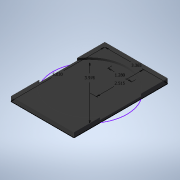
# Autodesk Inventor part: 100mm wafer wellplate
Saved by Autodesk Inventor 2020 (Build 240168000, 168)
## iProperties
Created: 2022-04-03
Part Number: 100mm wafer wellplate
Material: Generic
Document SubType Name: Modeling
Designer: Beaucage
Density: 1 g/cm^3
Appearance: Default
Author: Beaucage
Autodesk Inventor part; units mm, degrees
ref_plane "YZ Plane" through (0, 0, 0) normal (1, 0, 0) x (0, 1, 0)
ref_plane "XZ Plane" through (0, 0, 0) normal (0, 1, 0) x (-1, 0, 0)
ref_plane "XY Plane" through (0, 0, 0) normal (0, 0, 1) x (1, 0, 0)
sketch "Sketch1" plane through (0, 0, 0) normal (0, 1, 0) x (-1, 0, 0)
  line L0 (0, 0) -> (85.48, 0)
  line L1 (85.48, 0) -> (85.48, -127.76)
  line L2 (85.48, -127.76) -> (0, -127.76)
  line L3 (0, -127.76) -> (0, 0)
  line L4 (42.74, -127.76) -> (42.74, -63.879)
  circle A0 centre (42.1561, -63.879) radius 50.5
  line L5 (26.485, -111.163) -> (58.985, -111.1664)
  line L6 (42.74, -63.879) -> (42.7347, -113.879)
  point P0 (85.48, -37.9311)
  point P1 (85.48, -89.8269)
  point P2 (0, -91.6839)
  point P3 (0, -36.0741)
  point P4 (42.735, -111.1647)
  point P5 (42.74, -111.1647)
  point P6 (42.74, -114.3756)
  dimension "d0" = 85.48
  dimension "d1" = 127.76
  dimension "d2" = 63.881
  dimension "d3" = 101
  dimension "d4" = 32.5
  constraints: 14 end point, 3 perpendicular, 2 parallel, 2 point on circle, 2 point on line, 1 centre point, 1 coincident, 1 horizontal, 1 midpoint
  measures "d0" distance of L1.end L2.end
  measures "d1" distance of L0.end L1.end
  measures "d2" distance of L4.start L4.end
  measures "d3" diameter of A0
  measures "d4" distance of L5.start L5.end
extrude "Extrusion1" add sketch "Sketch1" along normal blind 6.35 contours L0 L1 A0 L3 | A0 L4 L2 L3 | L1 L2 L4 A0
extrude "Extrusion2" add sketch "Sketch1" along normal blind 3.175 contours L5 L6 L4 | A0 L1 L3
body "Solid1"
